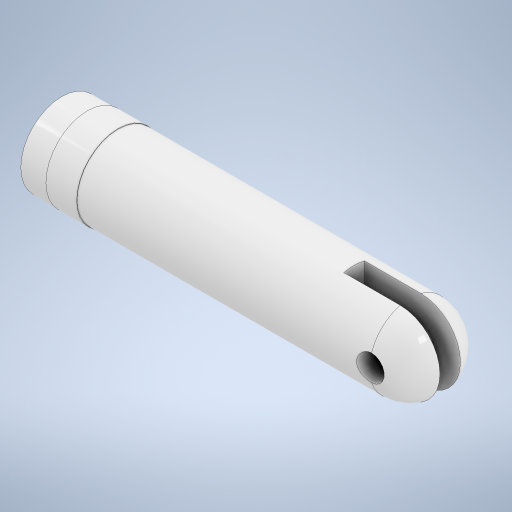
# Autodesk Inventor part: 1 -HUDSON-8-31B-TDR HAND PUMP
Saved by Autodesk Inventor 2024.2 (Build 282272000, 272)
## iProperties
Created: 2024-11-09
Part Number: 1 -HUDSON-8-31B-TDR HAND PUMP
Material: Genérico
Document SubType Name: Modeling
Designer: brene
Density: 1 g/cm^3
Appearance: Blanco
Author: brene
Autodesk Inventor part; units mm, degrees
ref_plane "YZ Plane" through (0, 0, 0) normal (1, 0, 0) x (0, 1, 0)
ref_plane "XZ Plane" through (0, 0, 0) normal (0, 1, 0) x (-1, 0, 0)
sketch "Boceto1" plane through (0, 0, 0) normal (0, 1, 0) x (-1, 0, 0)
  line L0 (52.4225, 0) -> (-52.4225, 0)
  line L1 (38.3374, 0) -> (38.3374, -8)
  line L2 (38.3374, -8) -> (-29.6626, -8)
  line L3 (-29.6626, -8) -> (-29.6626, 0)
  line L4 (38.3374, -5) -> (27.3374, -5)
  line L5 (27.3374, -5) -> (27.3374, 0)
  line L6 (33.3374, -8) -> (33.3374, -8.1)
  line L7 (33.3374, -8.1) -> (27.3374, -8.1)
  line L8 (27.3374, -8.1) -> (27.3374, -8)
  arc A0 (-37.6626, 0) -> (-29.6626, -8) centre (-29.6626, 0) ccw
  line L9 (-18.6626, 2) -> (-37.6626, 2)
  line L10 (-37.6626, 2) -> (-37.6626, -2)
  line L11 (-37.6626, -2) -> (-18.6626, -2)
  line L12 (-18.6626, -2) -> (-18.6626, 2)
  point P0 (0, 0)
  point P1 (0, 0)
  point P2 (-29.6626, -10)
  dimension "d0" = 68
  dimension "d1" = 16
  dimension "d2" = 10
  dimension "d3" = 11
  dimension "d4" = 5
  dimension "d5" = 6
  dimension "d6" = 16.2
  dimension "d8" = 8
  dimension "d9" = 19
  dimension "d10" = 4
  dimension "d11" = 10
  dimension "d12" = 38.3374
  dimension "d13" = 14.0851
  dimension "d14" = 68
  constraints: 26 end point, 7 point on line, 6 perpendicular, 3 horizontal, 2 coincident, 2 midpoint, 2 parallel, 2 point on circle, 2 vertical, 1 centre point
  measures "d0" distance of L2.end L1.end
  measures "d1" diameter of L2 L0
  measures "d2" diameter of L4 L0
  measures "d3" distance of L4.start L4.end
  measures "d4" distance of L1.end L6.start
  measures "d5" distance of L6.end L7.end
  measures "d6" diameter of L7 L0
  measures "d8" distance of A0.start L3.end
  measures "d9" distance of L10.end L11.end
  measures "d10" distance of L10.end L9.end
  measures "d11" vertical distance of A0.start point (-29.663, -10)
  measures "d12" distance from line of point (0, 0) L1
  measures "d13" distance from line of L0.start L1
  measures "d14" distance from line of point (-29.663, -10) L1
revolve "Revolución1" add sketch "Boceto1" angle 360 about axis through (-52.4225, 0, 0) along (1, 0, 0) contours L5 L4 L1 L2 L3 L11 L12 L0 | L12 L11 L3 L0 | L3 L11 A0 L0 | L6 L7 L8 L2 | L3 A0 L11
extrude "Extrusión1" cut sketch "Boceto1" along normal through all both and the other way through all contours L12 L11 L3 L0 | L0 L10 L9 L12 | L3 L11 A0 L0 | A0 L11 L10
ref_plane "Plano de trabajo1" through (29.6626, 0, -10) normal (0, 0, 1) x (1, 0, 0)
sketch "Boceto2" plane through (29.6626, 0, -10) normal (0, 0, 1) x (1, 0, 0)
  line L0 (-11, 7.746) -> (0, 7.746) projected
  line L1 (0, -7.746) -> (0, 7.746) projected
  line L2 (0, -7.746) -> (-11, -7.746) projected
  line L3 (-11, -7.746) -> (-11, -7.746) projected
  line L4 (-11, -7.746) -> (0, -7.746) projected
  line L5 (0, 7.746) -> (0, -7.746) projected
  line L6 (0, 7.746) -> (-11, 7.746) projected
  line L7 (-11, 7.746) -> (-11, 7.746) projected
  line L8 (-57, -8) -> (-57, 8) projected
  arc A0 (0, -7.746) -> (0, 7.746) centre (0, 0) ccw projected
  line L9 (0, -7.746) -> (0, 7.746) projected
  point P0 (-29.6626, 0)
  constraints: 1 coincident
hole "Agujero1" at (29.6626, 0, -10) direction (0, 0, 1) diameter 5 end through all
